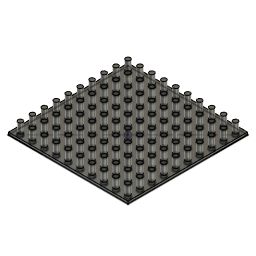
tippusher v1 (Autodesk Fusion 360 design; units mm, degrees)
Autodesk Fusion 360 part; units mm, degrees
sketch "Sketch1" plane through (0, 0, 0) normal (0, 0, 1) x (1, 0, 0)
  line L0 (100, 100) -> (-100, 100)
  line L1 (-100, 100) -> (-100, -100)
  line L2 (-100, -100) -> (100, -100)
  line L3 (100, -100) -> (100, 100)
  line L4 (100, 100) -> (-100, -100) construction
  line L5 (-100, 100) -> (100, -100) construction
  circle A0 centre (-90, -90) radius 4
  circle A1 centre (-70, -90) radius 4
  circle A2 centre (-50, -90) radius 4
  circle A3 centre (-30, -90) radius 4
  circle A4 centre (-10, -90) radius 4
  circle A5 centre (10, -90) radius 4
  circle A6 centre (30, -90) radius 4
  circle A7 centre (50, -90) radius 4
  circle A8 centre (70, -90) radius 4
  circle A9 centre (90, -90) radius 4
  circle A10 centre (-90, -70) radius 4
  circle A11 centre (-70, -70) radius 4
  circle A12 centre (-50, -70) radius 4
  circle A13 centre (-30, -70) radius 4
  circle A14 centre (-10, -70) radius 4
  circle A15 centre (10, -70) radius 4
  circle A16 centre (30, -70) radius 4
  circle A17 centre (50, -70) radius 4
  circle A18 centre (70, -70) radius 4
  circle A19 centre (90, -70) radius 4
  circle A20 centre (-90, -50) radius 4
  circle A21 centre (-70, -50) radius 4
  circle A22 centre (-50, -50) radius 4
  circle A23 centre (-30, -50) radius 4
  circle A24 centre (-10, -50) radius 4
  circle A25 centre (10, -50) radius 4
  circle A26 centre (30, -50) radius 4
  circle A27 centre (50, -50) radius 4
  circle A28 centre (70, -50) radius 4
  circle A29 centre (90, -50) radius 4
  circle A30 centre (-90, -30) radius 4
  circle A31 centre (-70, -30) radius 4
  circle A32 centre (-50, -30) radius 4
  circle A33 centre (-30, -30) radius 4
  circle A34 centre (-10, -30) radius 4
  circle A35 centre (10, -30) radius 4
  circle A36 centre (30, -30) radius 4
  circle A37 centre (50, -30) radius 4
  circle A38 centre (70, -30) radius 4
  circle A39 centre (90, -30) radius 4
  circle A40 centre (-90, -10) radius 4
  circle A41 centre (-70, -10) radius 4
  circle A42 centre (-50, -10) radius 4
  circle A43 centre (-30, -10) radius 4
  circle A44 centre (-10, -10) radius 4
  circle A45 centre (10, -10) radius 4
  circle A46 centre (30, -10) radius 4
  circle A47 centre (50, -10) radius 4
  circle A48 centre (70, -10) radius 4
  circle A49 centre (90, -10) radius 4
  circle A50 centre (-90, 10) radius 4
  circle A51 centre (-70, 10) radius 4
  circle A52 centre (-50, 10) radius 4
  circle A53 centre (-30, 10) radius 4
  circle A54 centre (-10, 10) radius 4
  circle A55 centre (10, 10) radius 4
  circle A56 centre (30, 10) radius 4
  circle A57 centre (50, 10) radius 4
  circle A58 centre (70, 10) radius 4
  circle A59 centre (90, 10) radius 4
  circle A60 centre (-90, 30) radius 4
  circle A61 centre (-70, 30) radius 4
  circle A62 centre (-50, 30) radius 4
  circle A63 centre (-30, 30) radius 4
  circle A64 centre (-10, 30) radius 4
  circle A65 centre (10, 30) radius 4
  circle A66 centre (30, 30) radius 4
  circle A67 centre (50, 30) radius 4
  circle A68 centre (70, 30) radius 4
  circle A69 centre (90, 30) radius 4
  circle A70 centre (-90, 50) radius 4
  circle A71 centre (-70, 50) radius 4
  circle A72 centre (-50, 50) radius 4
  circle A73 centre (-30, 50) radius 4
  circle A74 centre (-10, 50) radius 4
  circle A75 centre (10, 50) radius 4
  circle A76 centre (30, 50) radius 4
  circle A77 centre (50, 50) radius 4
  circle A78 centre (70, 50) radius 4
  circle A79 centre (90, 50) radius 4
  circle A80 centre (-90, 70) radius 4
  circle A81 centre (-70, 70) radius 4
  circle A82 centre (-50, 70) radius 4
  circle A83 centre (-30, 70) radius 4
  circle A84 centre (-10, 70) radius 4
  circle A85 centre (10, 70) radius 4
  circle A86 centre (30, 70) radius 4
  circle A87 centre (50, 70) radius 4
  circle A88 centre (70, 70) radius 4
  circle A89 centre (90, 70) radius 4
  circle A90 centre (-90, 90) radius 4
  circle A91 centre (-70, 90) radius 4
  circle A92 centre (-50, 90) radius 4
  circle A93 centre (-30, 90) radius 4
  circle A94 centre (-10, 90) radius 4
  circle A95 centre (10, 90) radius 4
  circle A96 centre (30, 90) radius 4
  circle A97 centre (50, 90) radius 4
  circle A98 centre (70, 90) radius 4
  circle A99 centre (90, 90) radius 4
  dimension "d1" = 200
  dimension "d2" = 200
  dimension "d3" = 8
  dimension "d4" = 10
  dimension "d7" = 180
  dimension "d8" = 180
  constraint perpendicular L0 L1
  constraint parallel L0 L2
  constraint parallel L1 L3
  constraint horizontal L0
  constraint coincident L4 origin
  constraint coincident L5 origin
  constraint coincident L4 A0.centre
  measures "d1" distance of L1.end L2.end
  measures "d2" distance of L0.end L1.end
  measures "d3" diameter of A0
  measures "d4" distance of L2 A0.centre
extrude "Extrude1" add sketch "Sketch1" along normal blind 20 contours A0 | A1 | A2 | A3 | A4 | A5 | A6 | A7 | A8 | A9 | A10 | A11 | A12 | A13 | A14 | A15 | A16 | A17 | A18 | A19 | A20 | A21 | A22 | A23 | A24 | A25 | A26 | A27 | A28 | A29 | A30 | A31 | A32 | A33 | A34 | A35 | A36 | A37 | A38 | A39 | A40 | A41 | A42 | A43 | A44 | A45 | A46 | A47 | A48 | A49 | A50 | A51 | A52 | A53 | A54 | A55 | A56 | A57 | A58 | A59 | A60 | A61 | A62 | A63 | A64 | A65 | A66 | A67 | A68 | A69 | A70 | A71 | A72 | A73 | A74 | A75 | A76 | A77 | A78 | A79 | A80 | A81 | A82 | A83 | A84 | A85 | A86 | A87 | A88 | A89 | A90 | A91 | A92 | A93 | A94 | A95 | A96 | A97 | A98 | A99 makes body 1 at (-66.005, 9.8006, 13.3333) makes body 2 at (-26.005, -50.1994, 13.3333) makes body 3 at (13.995, 29.8006, 13.3333) makes body 4 at (33.995, -70.1994, 13.3333) makes body 5 at (-86.005, -90.1994, 13.3333) makes body 6 at (-26.005, -90.1994, 13.3333) makes body 7 at (73.995, -70.1994, 13.3333) makes body 8 at (-86.005, 9.8006, 13.3333) makes body 9 at (-46.005, -90.1994, 13.3333) makes body 10 at (53.995, -70.1994, 13.3333) makes body 11 at (-86.005, -10.1994, 13.3333) makes body 12 at (-46.005, -10.1994, 13.3333) makes body 13 at (-6.005, 69.8006, 13.3333) makes body 14 at (-46.005, 69.8006, 13.3333) makes body 15 at (53.995, -50.1994, 13.3333) makes body 16 at (13.995, -10.1994, 13.3333) makes body 17 at (-66.005, -30.1994, 13.3333) makes body 18 at (-6.005, -30.1994, 13.3333) makes body 19 at (33.995, -50.1994, 13.3333) makes body 20 at (-26.005, 89.8006, 13.3333) makes body 21 at (73.995, 29.8006, 13.3333) makes body 22 at (93.995, -50.1994, 13.3333) makes body 23 at (33.995, 69.8006, 13.3333) makes body 24 at (-86.005, 69.8006, 13.3333) makes body 25 at (73.995, -10.1994, 13.3333) makes body 26 at (13.995, 69.8006, 13.3333) makes body 27 at (-26.005, 69.8006, 13.3333) makes body 28 at (93.995, 69.8006, 13.3333) makes body 29 at (-46.005, 49.8006, 13.3333) makes body 30 at (33.995, 49.8006, 13.3333) makes body 31 at (93.995, -10.1994, 13.3333) makes body 32 at (-66.005, 49.8006, 13.3333) makes body 33 at (93.995, 89.8006, 13.3333) makes body 34 at (13.995, -50.1994, 13.3333) makes body 35 at (93.995, 29.8006, 13.3333) makes body 36 at (53.995, -30.1994, 13.3333) makes body 37 at (-46.005, 89.8006, 13.3333) makes body 38 at (-6.005, 29.8006, 13.3333) makes body 39 at (-26.005, -10.1994, 13.3333) makes body 40 at (53.995, 29.8006, 13.3333) makes body 41 at (-6.005, -50.1994, 13.3333) makes body 42 at (73.995, 9.8006, 13.3333) makes body 43 at (-66.005, 29.8006, 13.3333) makes body 44 at (-66.005, -90.1994, 13.3333) makes body 45 at (73.995, -90.1994, 13.3333) makes body 46 at (-46.005, 9.8006, 13.3333) makes body 47 at (-6.005, -90.1994, 13.3333) makes body 48 at (-86.005, -70.1994, 13.3333) makes body 49 at (33.995, 29.8006, 13.3333) makes body 50 at (-26.005, 9.8006, 13.3333) makes body 51 at (-26.005, 29.8006, 13.3333) makes body 52 at (-46.005, 29.8006, 13.3333) makes body 53 at (-66.005, -70.1994, 13.3333) makes body 54 at (-46.005, -50.1994, 13.3333) makes body 55 at (53.995, 9.8006, 13.3333) makes body 56 at (-86.005, 29.8006, 13.3333) makes body 57 at (13.995, -70.1994, 13.3333) makes body 58 at (-26.005, -70.1994, 13.3333) makes body 59 at (-86.005, -50.1994, 13.3333) makes body 60 at (33.995, -90.1994, 13.3333) makes body 61 at (-66.005, -10.1994, 13.3333) makes body 62 at (53.995, -10.1994, 13.3333) makes body 63 at (73.995, 49.8006, 13.3333) makes body 64 at (33.995, 89.8006, 13.3333) makes body 65 at (-26.005, 49.8006, 13.3333) makes body 66 at (13.995, -30.1994, 13.3333) makes body 67 at (-66.005, 89.8006, 13.3333) makes body 68 at (73.995, -30.1994, 13.3333) makes body 69 at (-86.005, 49.8006, 13.3333) makes body 70 at (33.995, -30.1994, 13.3333) makes body 71 at (-26.005, -30.1994, 13.3333) makes body 72 at (-46.005, -30.1994, 13.3333) makes body 73 at (13.995, 89.8006, 13.3333) makes body 74 at (93.995, -30.1994, 13.3333) makes body 75 at (-6.005, 89.8006, 13.3333) makes body 76 at (-66.005, 69.8006, 13.3333) makes body 77 at (53.995, 49.8006, 13.3333) makes body 78 at (53.995, 89.8006, 13.3333) makes body 79 at (-86.005, 89.8006, 13.3333) makes body 80 at (73.995, 89.8006, 13.3333) makes body 81 at (93.995, 49.8006, 13.3333) makes body 82 at (73.995, 69.8006, 13.3333) makes body 83 at (-6.005, 49.8006, 13.3333) makes body 84 at (73.995, -50.1994, 13.3333) makes body 85 at (13.995, 49.8006, 13.3333) makes body 86 at (53.995, 69.8006, 13.3333) makes body 87 at (33.995, -10.1994, 13.3333) makes body 88 at (-86.005, -30.1994, 13.3333) makes body 89 at (-6.005, -10.1994, 13.3333) makes body 90 at (93.995, -70.1994, 13.3333) makes body 91 at (33.995, 9.8006, 13.3333) makes body 92 at (53.995, -90.1994, 13.3333) makes body 93 at (-66.005, -50.1994, 13.3333) makes body 94 at (-46.005, -70.1994, 13.3333) makes body 95 at (93.995, -90.1994, 13.3333) makes body 96 at (-6.005, 9.8006, 13.3333) makes body 97 at (-6.005, -70.1994, 13.3333) makes body 98 at (93.995, 9.8006, 13.3333) makes body 99 at (13.995, -90.1994, 13.3333) makes body 100 at (13.995, 9.8006, 13.3333)
extrude "Extrude2" add sketch "Sketch1" along normal blind 4 bodies 1 2 3 4 5 6 7 8 9 10 11 12 13 14 15 16 17 18 19 20 21 22 23 24 25 26 27 28 29 30 31 32 33 34 35 36 37 38 39 40 41 42 43 44 45 46 47 48 49 50 51 52 53 54 55 56 57 58 59 60 61 62 63 64 65 66 67 68 69 70 71 72 73 74 75 76 77 78 79 80 81 82 83 84 85 86 87 88 89 90 91 92 93 94 95 96 97 98 99 100
